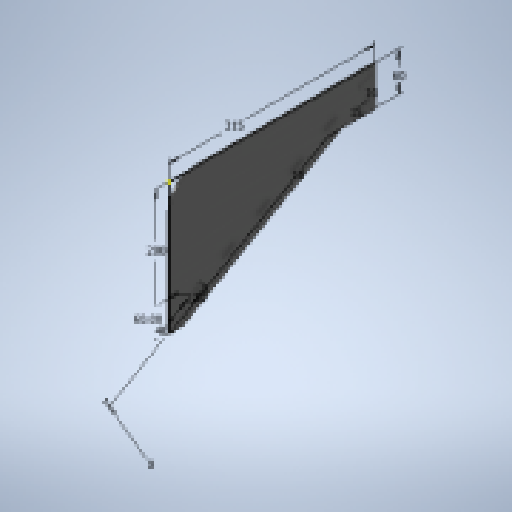
# Autodesk Inventor part: 2309HCMUTE-CDT23_VACH-NGAN
Saved by Autodesk Inventor 2023 (Build 270158000, 158)
## iProperties
Created: 2023-10-13
Part Number: 2309HCMUTE-CDT23_VACH-NGAN
Material: PMMA Plastic
Document SubType Name: Modeling
Designer: havie
Density: 1.188 g/cm^3
Appearance: Dark Gray
Author: havie
Autodesk Inventor part; units mm, degrees
ref_plane "YZ Plane" through (0, 0, 0) normal (1, 0, 0) x (0, 1, 0)
ref_plane "XZ Plane" through (0, 0, 0) normal (0, 1, 0) x (-1, 0, 0)
ref_plane "XY Plane" through (0, 0, 0) normal (0, 0, 1) x (1, 0, 0)
sketch "Sketch1" plane through (0, 0, 0) normal (1, 0, 0) x (0, 1, 0)
  line L0 (0, -315) -> (0, 0)
  line L1 (-60, -315) -> (0, -315)
  line L2 (-60, -315) -> (-60, -242.4871)
  line L3 (-60, -242.4871) -> (-200, 0)
  line L4 (-200, 0) -> (0, 0)
  line L5 (-177.4019, -33.141) -> (-167.4019, -50.4615)
  line L6 (-167.4019, -50.4615) -> (-170, -51.9615)
  line L7 (-170, -51.9615) -> (-180, -34.641)
  line L8 (-180, -34.641) -> (-177.4019, -33.141)
  line L9 (-200, -20) -> (-60, -262.4871)
  line L10 (-200, 0) -> (-200, -20)
  point P0 (-45, -305)
  point P1 (-175, -43.3013)
  point P2 (-172.4019, -41.8013)
  dimension "d0" = 60
  dimension "d7" = 15
  dimension "d47" = 315
  dimension "d48" = 200
  dimension "d49" = 60
  dimension "d51" = 3
  dimension "d52" = 20
  dimension "d54" = 40
  dimension "d59" = 10
  dimension "d60" = 0
  dimension "d63" = 10
  constraints: 22 end point, 4 perpendicular, 3 vertical, 2 midpoint, 1 coincident, 1 horizontal alignment, 1 parallel, 1 point on line
  measures "d0" distance of L1.start L0.start
  measures "d7" distance from line of L2 point (-45, -305)
  measures "d47" distance of L0.start L0.end
  measures "d48" distance of L3.end L0.end
  measures "d49" angle of L3 L4
  measures "d51" distance between parallel lines of L7 L5
  measures "d52" distance of L6.end L7.end
  measures "d54" distance from line of L3.end L8
  measures "d59" distance between parallel lines of L3 L9
  measures "d60" distance between parallel lines of L3 L7
  measures "d63" distance from line of L1 point (-45, -305)
extrude "Extrusion1" add sketch "Sketch1" along normal mid plane 3
sketch "Sketch2" plane through (1.5, 0, 0) normal (1, 0, 0) x (0, 0, -1)
  line L0 (29.641, -171.3397) -> (46.9615, -161.3397)
  line L1 (46.9615, -161.3397) -> (45.4615, -158.7417)
  line L2 (45.4615, -158.7417) -> (28.141, -168.7417)
  line L3 (28.141, -168.7417) -> (29.641, -171.3397)
  line L4 (0, 0) -> (0, -200) construction
  line L5 (20, -200) -> (262.4871, -60) projected
  dimension "d24" = 3
  dimension "d25" = 20
  dimension "d55" = 40
  dimension "d61" = 20
  constraints: 8 end point, 2 perpendicular, 1 parallel
  measures "d24" distance between parallel lines of L0 L2
  measures "d25" distance of L0.start L0.end
  measures "d55" distance from line of L4.end L3
  measures "d61" distance between parallel lines of L5 L0
extrude "Extrusion2" cut sketch "Sketch2" against normal blind 3
pattern_linear "Rectangular Pattern1" count 6 spacing 60 along (0, 0.5, -0.8660254) of "Extrusion2"
sketch "Sketch3" plane through (1.5, 0, 0) normal (1, 0, 0) x (0, 0, -1)
  line L0 (315, -60) -> (315, 0) projected
  line L1 (315, 0) -> (0, 0) projected
  line L2 (262.4871, -60) -> (315, -60) projected
  point P0 (300, -45)
  dimension "d64" = 15
  dimension "d65" = 15
  measures "d64" distance from line of L2 point (300, -45)
  measures "d65" distance from line of L0 point (300, -45)
hole "Hole3" at (1.5, -45, -300) direction (-1, 0, 0) diameter 4.134 end through all thread size "M5x0.8" class "6H" standard "ISO Metric profile"
fillet "Fillet1" radius 40 1 edges at (0, 0, 0)
body "Solid1"
